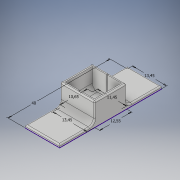
# Autodesk Inventor part: led_and_battery_holder
Saved by Autodesk Inventor 2019 (Build 230136000, 136)
## iProperties
Created: 2019-05-28
Part Number: led_and_battery_holder
Material: Generic
Document SubType Name: Modeling
Designer: assman
Density: 1 g/cm^3
Appearance: Default
Author: assman
## iProperties of the stored document led_and_battery_holder_3DPrint.ipt
Created: 2019-05-28
Part Number: led_and_battery_holder_3DPrint
Material: Generic
Document SubType Name: Modeling
Designer: assman
Density: 1 g/cm^3
Appearance: Default
Author: assman
Autodesk Inventor part; units mm, degrees
ref_plane "YZ Plane" through (0, 0, 0) normal (1, 0, 0) x (0, 1, 0)
ref_plane "XZ Plane" through (0, 0, 0) normal (0, 1, 0) x (-1, 0, 0)
ref_plane "XY Plane" through (0, 0, 0) normal (0, 0, 1) x (1, 0, 0)
sketch "Sketch1" plane through (0, 0, 0) normal (0, 1, 0) x (-1, 0, 0)
  line L0 (-5.725, 5.325) -> (5.725, 5.325)
  line L1 (5.725, 5.325) -> (5.725, -5.325)
  line L2 (5.725, -5.325) -> (-5.725, -5.325)
  line L3 (-5.725, -5.325) -> (-5.725, 5.325)
  line L4 (-5.725, 5.325) -> (5.725, -5.325) construction
  line L5 (5.725, 5.325) -> (-5.725, -5.325) construction
  line L6 (6.725, 20) -> (-6.725, 20)
  line L7 (-6.725, 20) -> (-6.725, -20)
  line L8 (-6.725, -20) -> (6.725, -20)
  line L9 (6.725, -20) -> (6.725, 20)
  line L10 (6.725, 20) -> (-6.725, -20) construction
  line L11 (-6.725, 20) -> (6.725, -20) construction
  line L12 (6.725, 6.275) -> (-6.725, 6.275)
  line L13 (-6.725, 6.275) -> (-6.725, -6.275)
  line L14 (-6.725, -6.275) -> (6.725, -6.275)
  line L15 (6.725, -6.275) -> (6.725, 6.275)
  line L16 (6.725, 6.275) -> (-6.725, -6.275) construction
  line L17 (-6.725, 6.275) -> (6.725, -6.275) construction
  point P0 (0, 0)
  dimension "d0" = 11.45
  dimension "d1" = 10.65
  dimension "d2" = 13.45
  dimension "d3" = 40
  dimension "d4" = 12.55
  dimension "d5" = 13.45
  constraints: 36 end point, 6 midpoint, 6 parallel, 3 horizontal, 3 perpendicular
  measures "d0" distance of L1.end L2.end
  measures "d1" distance of L0.end L1.end
  measures "d2" distance of L8.end L7.end
  measures "d3" distance of L8.end L6.start
  measures "d4" distance of L13.end L12.end
  measures "d5" distance of L12.start L12.end
extrude "Extrusion1" add sketch "Sketch1" along normal blind 1 contours L9 L12 L7 L6 | L9 L8 L7 L14
extrude "Extrusion2" add sketch "Sketch1" along normal blind 8.725 contours L9 L14 L7 L12
extrude "Extrusion3" add sketch "Sketch1" along normal blind 1 contours L0 L1 L2 L3
fillet "Fillet1" radius 2 2 edges at (5.725, 1, 0) (-5.725, 1, 0)
fillet "Fillet2" radius 2 2 edges at (0, 1, -6.275) (0, 1, 6.275)
fillet "Fillet3" radius 0.5 18 edges at (-6.725, 1.5858, -6.8608) (-6.725, 1, -14.1375) (-6.725, 5.8625, -6.275) (6.725, 1.5858, -6.8608) (6.725, 1, -14.1375) (6.725, 5.8625, -6.275) (0, 1, -20) (0, 1, 20) (-6.725, 1.5858, 6.8608) (-6.725, 5.8625, 6.275) (-6.725, 1, 14.1375) (6.725, 5.8625, 6.275) (6.725, 1, 14.1375) (6.725, 1.5858, 6.8608) (-6.725, 8.725, 0) (0, 8.725, -6.275) (6.725, 8.725, 0) (0, 8.725, 6.275)
sketch "Sketch2" plane through (5.725, 8.725, 5.325) normal (0, 0, -1) x (-1, 0, 0)
  arc A0 (9.45, -7.725) -> (11.45, -5.725) centre (9.45, -5.725) ccw construction
  line L0 (11.45, -5.725) -> (11.45, 0) construction
  line L1 (0, 0) -> (11.45, 0) construction
  line L2 (0, -5.725) -> (0, 0) construction
  arc A1 (0, -5.725) -> (2, -7.725) centre (2, -5.725) ccw construction
  line L3 (2, -7.725) -> (9.45, -7.725) construction
  circle A2 centre (5.725, -1.725) radius 5.725
  point P0 (5.725, -8.725)
  dimension "d15" = 11.45
  dimension "d16" = 6
  constraints: 1 centre point
  measures "d15" diameter of A2
  measures "d16" distance from line of L3 A2.centre
extrude "Extrusion4" add sketch "Sketch2" along normal blind 10.55 separate body
sketch "Sketch3" plane through (0, 1, 0) normal (0, 1, 0) x (1, 0, 0)
  line L0 (-3.725, -5.325) -> (-3.725, 5.325) construction
  line L1 (3.725, -5.325) -> (-3.725, -5.325) construction
  line L2 (3.725, 5.325) -> (3.725, -5.325) construction
  line L3 (-3.725, 5.325) -> (3.725, 5.325) construction
  line L4 (-0.225, -5.775) -> (0.225, -5.775)
  line L5 (0.225, -5.775) -> (0.225, -5.325)
  line L6 (0.225, -5.325) -> (-0.225, -5.325)
  line L7 (-0.225, -5.325) -> (-0.225, -5.775)
  line L8 (-0.225, -5.775) -> (0.225, -5.325) construction
  line L9 (0.225, -5.775) -> (-0.225, -5.325) construction
  line L10 (0, -5.325) -> (0, 5.325) construction
  line L11 (-3.725, -5.325) -> (-3.725, 5.325) construction
  line L12 (-3.725, -5.325) -> (3.725, -5.325) construction
  line L13 (-3.725, 5.325) -> (3.725, 5.325) construction
  line L14 (-5.725, 5.325) -> (5.725, 5.325) construction
  line L15 (5.725, -5.325) -> (-5.725, -5.325) construction
  line L16 (-3.725, 0) -> (3.725, 0) construction
  line L17 (-0.225, 5.775) -> (0.225, 5.775)
  line L18 (0.225, 5.775) -> (0.225, 5.325)
  line L19 (0.225, 5.325) -> (-0.225, 5.325)
  line L20 (-0.225, 5.325) -> (-0.225, 5.775)
  point P0 (0, 0)
  point P1 (0, -5.55)
  point P2 (0, -5.55)
  dimension "d19" = 0.45
  dimension "d20" = 0.45
  constraints: 28 end point, 7 midpoint, 4 symmetric about line, 2 collinear, 2 parallel, 2 perpendicular, 1 horizontal, 1 point on line
  measures "d19" distance of L6.end L5.end
  measures "d20" distance of L5.end L4.end
extrude "Extrusion5" cut sketch "Sketch3" along normal blind 10 bodies 1
body "Solid1"
body "Solid2"
